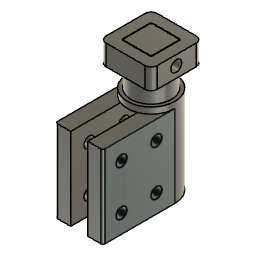
Fahnen_Halter v12 (Autodesk Fusion 360 design; units mm, degrees)
Autodesk Fusion 360 part; units mm, degrees
note: some values were not read from the file. Set by a fixed rule: which sketch regions a step uses.
sketch "Skizze1" plane through (0, 0, 0) normal (0, 0, 1) x (1, 0, 0)
  line L0 (18.25, 16) -> (18.25, 51)
  line L1 (18.25, 51) -> (9.95, 51)
  line L2 (9.95, 51) -> (9.95, 16)
  line L3 (9.95, 16) -> (2.55, 16)
  line L4 (2.55, 16) -> (2.55, 51)
  line L5 (9.95, 51) -> (18.25, 51)
  line L6 (25.65, 51) -> (25.65, 16)
  line L7 (25.65, 16) -> (18.25, 16)
  arc A0 (25.65, 51) -> (2.55, 51) centre (14.1, 51) ccw
  dimension "d1" = 8.3
  dimension "d2" = 7.4
  dimension "d3" = 7.4
  dimension "d4" = 35
  dimension "d36" = 11.55
  constraint vertical L0
  constraint perpendicular L0 L1
  constraint perpendicular L1 L2
  constraint perpendicular L0 L3
  constraint perpendicular L1 L4
  constraint perpendicular L4 L5
  constraint perpendicular L1 L6
  constraint perpendicular L0 L7
  constraint tangent L6 A0
  constraint collinear L3 L7
  constraint midpoint L1 A0.centre
  measures "d1" distance of L0.end L1.end
  measures "d2" distance of L2.end L3.end
  measures "d3" distance of L0 L6
  measures "d4" distance of L1.end L2.end
  measures "d36" radius of A0
extrude "Extrusion1" add sketch "Skizze1" along normal blind 40 makes body 1
sketch "Skizze2" plane through (25.65, 0, 0) normal (1, 0, 0) x (0, 1, 0)
  line L0 (16, 0) -> (51, 0)
  line L1 (51, 0) -> (51, 40)
  line L2 (51, 40) -> (16, 40)
  line L3 (16, 40) -> (16, 0)
  circle A0 centre (25, 31) radius 2.6
  circle A1 centre (42, 31) radius 2.6
  circle A2 centre (25, 9) radius 2.6
  circle A3 centre (42, 9) radius 2.6
  dimension "d7" = 5.2
  dimension "d8" = 9
  dimension "d9" = 9
  dimension "d10" = 5.2
  dimension "d11" = 9
  dimension "d12" = 9
  dimension "d13" = 5.2
  dimension "d14" = 5.2
  dimension "d15" = 9
  dimension "d16" = 9
  dimension "d17" = 9
  dimension "d18" = 9
  measures "d7" diameter of A0
  measures "d8" distance of L3 A0.centre
  measures "d9" distance of L1 A1.centre
  measures "d10" diameter of A1
  measures "d11" distance of L2 A1.centre
  measures "d12" distance of L2 A0.centre
  measures "d13" diameter of A2
  measures "d14" diameter of A3
  measures "d15" distance of L3 A2.centre
  measures "d16" distance of L0 A2.centre
  measures "d17" distance of L0 A3.centre
  measures "d18" distance of L1 A3.centre
extrude "Extrusion2" cut sketch "Skizze2" against normal up to surface (23.1 mm away) contours A0 | A1 | A2 | A3 bodies 1
sketch "Skizze3" plane through (0, 0, 40) normal (0, 0, 1) x (-1, 0, 0)
  line L0 (-25.65, -16) -> (-25.65, -51)
  arc A0 (-25.65, -51) -> (-2.55, -51) centre (-14.1, -51) ccw
  line L1 (-2.55, -51) -> (-2.55, -16)
  line L2 (-2.55, -16) -> (-9.95, -16)
  line L3 (-9.95, -16) -> (-9.95, -51)
  line L4 (-9.95, -51) -> (-18.25, -51)
  line L5 (-18.25, -51) -> (-18.25, -16)
  line L6 (-18.25, -16) -> (-25.65, -16)
  circle A1 centre (-14.1, -51) radius 11.55
  constraint concentric A0 A1
  constraint tangent A0 A1
extrude "Extrusion6" add sketch "Skizze3" along normal blind 3 contours A0 L3 L4 L5 A1 | L3 L4 L5 A1 bodies 1
sketch "Skizze7" plane through (0, 0, 43) normal (0, 0, 1) x (-1, 0, 0)
  circle A0 centre (-14.1, -51) radius 11.55
  circle A1 centre (-14.1, -51) radius 9.85
  dimension "d39" = 19.7
  constraint concentric A0 A1
  measures "d39" diameter of A1
extrude "Extrusion7" add sketch "Skizze7" along normal blind 10.3 contours A1 bodies 1
sketch "Skizze5" plane through (0, 0, 53.3) normal (0, 0, 1) x (-1, 0, 0)
  circle A0 centre (-14.1, -51) radius 9.85
  line L0 (-21.065, -57.965) -> (-7.135, -57.965)
  line L1 (-7.135, -57.965) -> (-7.135, -44.035)
  line L2 (-7.135, -44.035) -> (-21.065, -44.035)
  line L3 (-21.065, -44.035) -> (-21.065, -57.965)
  line L4 (-21.065, -57.965) -> (-7.135, -44.035) construction
  line L5 (-7.135, -57.965) -> (-21.065, -44.035) construction
  line L6 (-6.885, -43.785) -> (-21.315, -43.785)
  line L7 (-21.315, -43.785) -> (-21.315, -58.215)
  line L8 (-21.315, -58.215) -> (-6.885, -58.215)
  line L9 (-6.885, -58.215) -> (-6.885, -43.785)
  line L10 (-26.565, -63.465) -> (-1.635, -63.465)
  line L11 (-1.635, -63.465) -> (-1.635, -38.535)
  line L12 (-1.635, -38.535) -> (-26.565, -38.535)
  line L13 (-26.565, -38.535) -> (-26.565, -63.465)
  point P0 (-14.1, -51)
  point P1 (-14.1, -51)
  dimension "d48" = 0.25
  dimension "d49" = 5.5
  constraint coincident P0 A0.centre
  constraint horizontal L0
  constraint perpendicular L0 L1
  constraint parallel L0 L2
  constraint parallel L1 L3
  constraint coincident L4 P1
  constraint coincident L5 P1
  constraint coincident P1 P0
  constraint equal L0 L3
  constraint coincident A0 L0.start
extrude "Extrusion8" add sketch "Skizze5" along normal blind 10 contours L0 L1 L2 L3 bodies 1
sketch "Skizze6" plane through (21.065, 0, 0) normal (1, 0, 0) x (0, 1, 0)
  line L0 (59.0964, 53.5) -> (59.0964, 63.5)
  line L1 (59.0964, 63.5) -> (42.9036, 63.5)
  line L2 (42.9036, 63.5) -> (42.9036, 53.5)
  circle A0 centre (50.7879, 58.5) radius 2.65
  line L3 (45.5676, 53.5) -> (56.4324, 53.5)
  line L4 (56.4324, 53.5) -> (59.0964, 53.5)
  line L5 (42.9036, 53.5) -> (45.5676, 53.5)
  line L6 (44.035, 53.3) -> (57.965, 53.3)
  line L7 (57.965, 53.3) -> (57.965, 63.3)
  line L8 (57.965, 63.3) -> (44.035, 63.3)
  line L9 (44.035, 63.3) -> (44.035, 53.3)
  dimension "d25" = 5.3
  dimension "d27" = 7.8842
  dimension "d28" = 7.8842
  dimension "d29" = 5
  measures "d25" diameter of A0
  measures "d27" distance of L2 A0.centre
  measures "d29" distance of L1 A0.centre
fillet "Abrundung1" radius 1 4 edges at (21.065, 57.965, 58.3) (21.065, 44.035, 58.3) (7.135, 44.035, 58.3) (7.135, 57.965, 58.3) on bodies 1
fillet "Abrundung2" radius 1 2 edges at (25.65, 16, 20) (2.55, 16, 20) on bodies 1
extrude "Extrusion9" add sketch "Skizze5" along normal blind 10 separate body contours A0 L9 | A0 L6 | A0 L8 | A0 L7 | L10 L11 L12 L13 makes body 2
fillet "Abrundung3" radius 0.6 4 edges at (21.315, 43.785, 58.3) (6.885, 43.785, 58.3) (6.885, 58.215, 58.3) (21.315, 58.215, 58.3) on bodies 2
extrude "Extrusion5" cut sketch "Skizze6" along normal blind -24 and the other way blind -12 contours A0 bodies 1 2
fillet "Abrundung4" radius 3 4 edges at (1.635, 38.535, 58.3) (26.565, 38.535, 58.3) (26.565, 63.465, 58.3) (1.635, 63.465, 58.3) on bodies 2
equation "d3 = d2"
equation "d10 = d7"
equation "d11 = d12"
equation "d14 = d7"
equation "d15 = d8"
equation "d16 = d12"
equation "d17 = d12"
equation "d18 = d9"
equation "d36 = d2 + d1 / 2"
